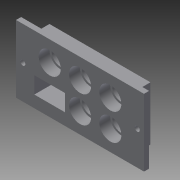
# Autodesk Inventor part: 5 led mount idea
Saved by Autodesk Inventor 2014 SP1 (Build 180222100, 222)
## iProperties
Created: 2017-07-19
Part Number: 5 led mount idea
Material: Generic
Document SubType Name: Modeling
Designer: kteo17
Density: 1 g/cm^3
Appearance: Default
Author: kteo17
Autodesk Inventor part; units mm, degrees
ref_plane "YZ Plane" through (0, 0, 0) normal (1, 0, 0) x (0, 1, 0)
ref_plane "XZ Plane" through (0, 0, 0) normal (0, 1, 0) x (-1, 0, 0)
ref_plane "XY Plane" through (0, 0, 0) normal (0, 0, 1) x (1, 0, 0)
sketch "Sketch1" plane through (0, 0, 0) normal (0, 0, 1) x (1, 0, 0)
  line L0 (0, 0) -> (47.625, 0)
  line L1 (47.625, 0) -> (47.625, 25.4)
  line L2 (47.625, 25.4) -> (0, 25.4)
  line L3 (0, 25.4) -> (0, 0)
  circle A0 centre (38.1, 6.35) radius 5.207
  circle A1 centre (23.8125, 6.35) radius 5.207
  circle A2 centre (23.8125, 19.05) radius 5.207
  circle A3 centre (38.1, 19.05) radius 5.207
  circle A4 centre (9.525, 19.05) radius 5.207
  line L4 (2.2603, 10.287) -> (16.7383, 10.287)
  line L5 (16.7383, 10.287) -> (16.7383, 2.413)
  line L6 (16.7383, 2.413) -> (2.2603, 2.413)
  line L7 (2.2603, 2.413) -> (2.2603, 10.287)
  line L8 (-6.35, 28.575) -> (53.975, 28.575)
  line L9 (53.975, 28.575) -> (53.975, -3.175)
  line L10 (53.975, -3.175) -> (-6.35, -3.175)
  line L11 (-6.35, -3.175) -> (-6.35, 28.575)
  dimension "d0" = 47.625
  dimension "d1" = 25.4
  dimension "d2" = 10.414
  dimension "d3" = 10.414
  dimension "d4" = 10.414
  dimension "d5" = 10.414
  dimension "d6" = 10.414
  dimension "d9" = 14.478
  dimension "d10" = 7.874
  dimension "d27" = 60.325
  dimension "d28" = 31.75
  constraints: 24 end point, 6 parallel, 5 centre point, 3 horizontal, 3 perpendicular
  measures "d0" distance of L2.end L1.end
  measures "d1" distance of L1.end L0.end
  measures "d2" diameter of A0
  measures "d3" diameter of A1
  measures "d4" diameter of A2
  measures "d5" diameter of A3
  measures "d6" diameter of A4
  measures "d9" distance of L5.end L6.end
  measures "d10" distance of L4.end L5.end
  measures "d27" distance of L8.start L8.end
  measures "d28" distance of L8.end L9.end
extrude "Extrusion1" add sketch "Sketch1" against normal blind 9.398 contours L3 L2 L1 L0 | L8 L9 L10 L11
sketch "Sketch3" plane through (0, 0, -9.398) normal (0, 0, -1) x (-1, 0, 0)
  line L0 (6.35, 28.575) -> (-53.975, 28.575) projected
  line L1 (-53.975, 28.575) -> (-53.975, -3.175) projected
  line L2 (-53.975, -3.175) -> (6.35, -3.175) projected
  line L3 (6.35, -3.175) -> (6.35, 28.575) projected
  line L4 (-47.625, 25.4) -> (0, 25.4)
  line L5 (0, 25.4) -> (0, 0)
  line L6 (0, 0) -> (-47.625, 0)
  line L7 (-47.625, 0) -> (-47.625, 25.4)
  constraints: 8 end point, 2 parallel, 1 horizontal, 1 perpendicular
extrude "Extrusion2" cut sketch "Sketch3" against normal blind 7.0104
sketch "Sketch4" plane through (0, 0, -9.398) normal (0, 0, -1) x (-1, 0, 0)
  circle A0 centre (-9.525, 19.05) radius 5.207 projected
  circle A1 centre (-38.1, 19.05) radius 5.207 projected
  circle A2 centre (-23.8125, 19.05) radius 5.207 projected
  circle A3 centre (-23.8125, 6.35) radius 5.207 projected
  circle A4 centre (-38.1, 6.35) radius 5.207 projected
  circle A5 centre (-38.1, 19.05) radius 4.191
  circle A6 centre (-23.8125, 19.05) radius 4.191
  circle A7 centre (-9.525, 19.05) radius 4.191
  circle A8 centre (-38.1, 6.35) radius 4.191
  circle A9 centre (-23.8125, 6.35) radius 4.191
  dimension "d17" = 8.382
  constraints: 5 centre point, 5 coincident
  measures "d17" diameter of A5
extrude "Extrusion3" add sketch "Sketch4" against normal blind 4.318
sketch "Sketch5" plane through (0, 0, -9.398) normal (0, 0, -1) x (-1, 0, 0)
  line L0 (-2.2603, 10.287) -> (-2.2603, 2.413) projected
  line L1 (-2.2603, 2.413) -> (-16.7383, 2.413) projected
  line L2 (-16.7383, 2.413) -> (-16.7383, 10.287) projected
  line L3 (-16.7383, 10.287) -> (-2.2603, 10.287) projected
  line L4 (-16.7383, 6.35) -> (-12.8013, 10.287)
  line L5 (-16.7383, 6.35) -> (-11.1705, 6.35) construction
  line L6 (-16.7383, 6.35) -> (-12.8013, 2.413)
  line L7 (-2.2603, 6.35) -> (-6.1973, 10.287)
  line L8 (-2.2603, 6.35) -> (-6.1973, 2.413)
  dimension "d20" = 45
  constraints: 10 end point, 4 point on line, 2 midpoint, 2 perpendicular, 1 equal length, 1 horizontal, 1 parallel
  measures "d20" angle of L5 L4
extrude "Extrusion4" add sketch "Sketch5" against normal blind 0.889 contours L0 L7 L3 | L0 L1 L8 | L4 L2 L3 | L1 L2 L6
sketch "Sketch6" plane through (0, 0, 0) normal (0, 0, 1) x (1, 0, 0)
  circle A0 centre (-3.175, 12.7) radius 1.1938
  circle A1 centre (50.8, 12.7) radius 1.1938
  point P0 (0, 0)
  dimension "d23" = 2.3876
  dimension "d24" = 2.3876
  constraints: 2 centre point
  measures "d23" diameter of A0
  measures "d24" diameter of A1
extrude "Extrusion5" cut sketch "Sketch6" against normal blind 2.3876
body "Solid1"
